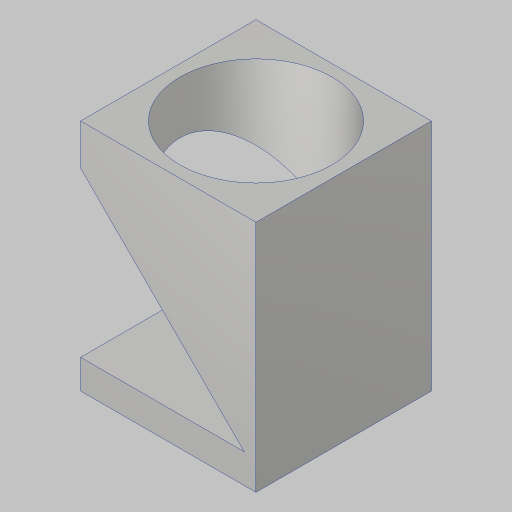
# Autodesk Inventor part: NoodleJig
Saved by Autodesk Inventor 2023.5 (Build 275446000, 446)
## iProperties
Created: 2025-03-08
Part Number: NoodleJig
Material: Aluminum 6061
Document SubType Name: Modeling
Designer: slick
Density: 2.7 g/cm^3
Appearance: Aluminum - Flat
Author: slick
Autodesk Inventor part; units mm, degrees
ref_plane "YZ Plane" through (0, 0, 0) normal (1, 0, 0) x (0, 1, 0)
ref_plane "XZ Plane" through (0, 0, 0) normal (0, 1, 0) x (-1, 0, 0)
ref_plane "XY Plane" through (0, 0, 0) normal (0, 0, 1) x (1, 0, 0)
sketch "Sketch1" plane through (0, 0, 0) normal (0, 1, 0) x (-1, 0, 0)
  line L0 (-38.1, 38.1) -> (38.1, 38.1)
  line L1 (38.1, 38.1) -> (38.1, -38.1)
  line L2 (38.1, -38.1) -> (-38.1, -38.1)
  line L3 (-38.1, -38.1) -> (-38.1, 38.1)
  line L4 (-38.1, 38.1) -> (38.1, -38.1) construction
  line L5 (38.1, 38.1) -> (-38.1, -38.1) construction
  point P0 (0, 0)
  dimension "d0" = 76.2
  dimension "d1" = 76.2
  constraints: 12 end point, 2 midpoint, 2 parallel, 1 horizontal, 1 perpendicular
  measures "d0" distance of L1.end L2.end
  measures "d1" distance of L0.end L1.end
extrude "Extrusion1" add sketch "Sketch1" along normal blind 101.6
sketch "Sketch2" plane through (0, 101.6, 0) normal (0, 1, 0) x (1, 0, 0)
  circle A0 centre (0, 0) radius 33.02
  dimension "d4" = 66.04
  constraints: 1 centre point, 1 coincident
  measures "d4" diameter of A0
extrude "Extrusion2" cut sketch "Sketch2" against normal blind 88.9
sketch "Sketch3" plane through (-38.1, 0, 38.1) normal (0, 0, 1) x (1, 0, 0)
  line L0 (0, 0) -> (0, 101.6) construction
  line L1 (0, 101.6) -> (76.2, 101.6) construction
  line L2 (76.2, 101.6) -> (76.2, 0) construction
  line L3 (76.2, 0) -> (0, 0) construction
  line L4 (0, 0) -> (0, 101.6) construction
  line L5 (0, 101.6) -> (76.2, 101.6) construction
  line L6 (76.2, 101.6) -> (76.2, 0) construction
  line L7 (76.2, 0) -> (0, 0) construction
  line L8 (5.08, 12.7) -> (71.12, 12.7) construction
  line L9 (5.08, 101.6) -> (71.12, 101.6) construction
  line L10 (5.08, 12.7) -> (71.12, 12.7) construction
  line L11 (71.12, 12.7) -> (0, 12.7)
  line L12 (0, 0) -> (0, 101.6) construction
  line L13 (71.12, 12.7) -> (0, 83.82)
  line L14 (0, 12.7) -> (0, 83.82)
  line L15 (0, 0) -> (0, 101.6) construction
  point P0 (38.1, 0)
  dimension "d7" = 45
  constraints: 6 end point, 2 point on line, 1 collinear, 1 horizontal
  measures "d7" angle of L13 L8
extrude "Extrusion3" cut sketch "Sketch3" against normal through all
body "Solid1"
